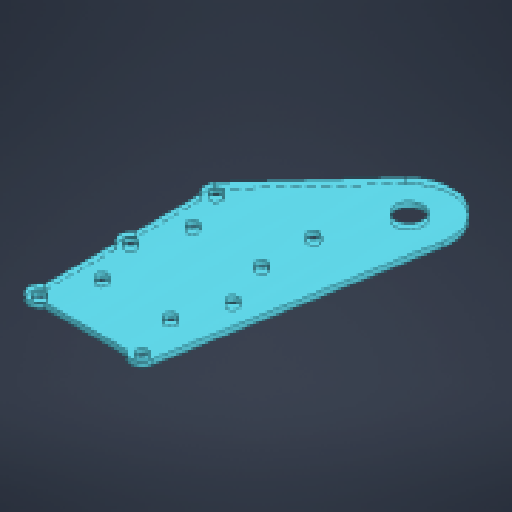
# Autodesk Inventor part: femur_support_steel
Saved by Autodesk Inventor 2026 (Build 300175000, 175)
## iProperties
Created: 2026-04-24
Part Number: femur_support_steel
Material: Сталь
Document SubType Name: Modeling
Designer: user
Density: 7.85 g/cm^3
Appearance: Серо-синий
Mass: 237.917 g
Surface Area: 222.677 cm^2
Volume: 30.3078 cm^3
Author: user
Autodesk Inventor part; units mm, degrees
ref_plane "YZ Plane" through (0, 0, 0) normal (1, 0, 0) x (0, 1, 0)
ref_plane "XZ Plane" through (0, 0, 0) normal (0, 1, 0) x (-1, 0, 0)
ref_plane "XY Plane" through (0, 0, 0) normal (0, 0, 1) x (1, 0, 0)
sketch "Эскиз1" plane through (0, 0, 0) normal (0, 1, 0) x (-1, 0, 0)
  circle A0 centre (41.8656, -145.8142) radius 7.75
  line L0 (111.6413, -108.8142) -> (38.7953, -108.8142) construction
  line L1 (76.8656, 21.9817) -> (76.8656, -112.0617)
  circle A1 centre (48.8156, -8.8142) radius 3.05
  circle A2 centre (57.9156, -33.8142) radius 3.05
  circle A3 centre (48.8156, -58.8142) radius 3.05
  circle A4 centre (57.9156, -83.8142) radius 3.05
  circle A5 centre (95.8156, -83.8142) radius 3.05
  circle A6 centre (104.9156, -58.8142) radius 3.05
  circle A7 centre (95.8156, -33.8142) radius 3.05
  circle A8 centre (104.9156, -8.8142) radius 3.05
  arc A9 (54.0984, -5.7642) -> (42.7519, -8.1498) centre (48.8156, -8.8142) ccw
  arc A10 (107.9656, -14.0969) -> (99.6329, -5.7642) centre (104.9156, -8.8142) ccw
  arc A11 (107.9656, -64.0969) -> (107.9656, -53.5314) centre (104.9156, -58.8142) ccw
  line L2 (107.9656, -102.9344) -> (107.9656, -64.0969)
  line L3 (107.9656, -53.5314) -> (107.9656, -14.0969)
  line L4 (99.6329, -5.7642) -> (54.0984, -5.7642)
  line L5 (32.6597, -100.2644) -> (42.7519, -8.1498)
  circle A12 centre (41.8656, -145.8142) radius 15 construction
  line L6 (101.8656, -108.8142) -> (101.8656, -72.3334) construction
  line L7 (101.8656, -108.8142) -> (26.8312, -181.1395) construction
  line L8 (51.8656, -108.8142) -> (51.8656, -72.3334) construction
  line L9 (95.7259, -114.7322) -> (107.9656, -102.9344)
  line L10 (95.7259, -114.7322) -> (98.5019, -117.6122)
  arc A13 (98.4405, -120.4492) -> (98.5019, -117.6122) centre (97.0619, -119.0002) ccw
  circle A14 centre (41.8656, -145.8142) radius 45 construction
  circle A15 centre (77.839, -118.7786) radius 5.05
  circle A16 centre (5.8923, -172.8497) radius 5.05
  arc A17 (-4.5085, -167.9431) -> (7.7127, -184.2047) centre (5.8923, -172.8497) ccw
  line L11 (-4.5085, -167.9431) -> (12.4721, -131.9479)
  line L12 (26.8312, -181.1395) -> (30.2073, -177.8853)
  line L13 (32.4723, -180.2351) -> (30.2073, -177.8853)
  arc A18 (47.0104, -177.9044) -> (71.2591, -159.6804) centre (41.8656, -145.8142) ccw
  arc A19 (21.5713, -120.4293) -> (12.4721, -131.9479) centre (41.8656, -145.8142) ccw
  line L14 (98.4405, -120.4492) -> (86.4967, -131.9617)
  line L15 (71.2591, -159.6804) -> (80.184, -140.7616)
  arc A20 (21.5713, -120.4293) -> (32.6597, -100.2644) centre (2.8381, -96.9971) ccw
  line L16 (7.7127, -184.2047) -> (26.8312, -181.1395)
  line L17 (32.4723, -180.2351) -> (47.0104, -177.9044)
  arc A21 (86.4967, -131.9617) -> (80.184, -140.7616) centre (107.3164, -153.5612) ccw
  point P0 (0, 0)
  point P1 (99.8898, -119.0521)
  point P2 (31.026, -115.1751)
  point P3 (82.5329, -135.7824)
  dimension "d4" = 37.9
  dimension "d5" = 56.1
  dimension "d6" = 6.1
  dimension "d7" = 50
  dimension "d8" = 50
  dimension "d9" = 25
  dimension "d10" = 50
  dimension "d11" = 37.9
  dimension "d12" = 56.1
  dimension "d15" = 35
  dimension "d16" = 37
  dimension "d17" = 15.5
  dimension "d20" = 12.2
  dimension "d21" = 12.2
  dimension "d24" = 3.05
  dimension "d26" = 30
  dimension "d29" = 50
  dimension "d33" = 10.1
  dimension "d36" = 360
  dimension "d38" = 90
  dimension "d40" = 9.5
  dimension "d42" = 32.5
  dimension "d44" = 23
  dimension "d45" = 6
  dimension "d47" = 11.5
  dimension "d48" = 30
  dimension "d49" = 17
  dimension "d50" = 91
  dimension "d51" = 30
  constraints: 36 end point, 21 centre point, 19 point on circle, 15 tangent, 11 point on line, 9 equal radius, 7 coincident, 4 horizontal alignment, 4 perpendicular, 4 vertical alignment, 2 symmetric about line, 2 vertical, 1 horizontal, 1 parallel, 9 other
  measures "d4" distance of A5.centre A4.centre
  measures "d5" distance of A8.centre A1.centre
  measures "d6" diameter of A1
  measures "d7" distance from line of A3.centre L0
  measures "d8" distance of A1.centre A3.centre
  measures "d9" distance from line of L0 A4.centre
  measures "d10" distance of A2.centre A4.centre
  measures "d11" diameter of A2.centre L1
  measures "d12" diameter of A1.centre L1
  measures "d15" distance from line of A0.centre L1
  measures "d16" distance from line of L0 A0.centre
  measures "d17" diameter of A0
  measures "d20" diameter of A10
  measures "d21" diameter of A11
  measures "d24" distance from line of L4 A8.centre
  measures "d26" diameter of A12
  measures "d29" diameter of L6 L1
  measures "d33" diameter of A15
  measures "d38" distance of A16.centre A15.centre
  measures "d40" distance from line of L7 A15.centre
  measures "d42" radius of A19
  measures "d44" diameter of A17
  measures "d45" distance between parallel lines of L14 L7
  measures "d47" distance from line of L15 A15.centre
  measures "d48" radius of A20
  measures "d49" distance from line of L10 L2.start
  measures "d50" distance between parallel lines of L10 L13
  measures "d51" radius of A21
extrude "Выдавливание1" add sketch "Эскиз1" along normal blind 3
equation "\"d4\" = -d_main_screw_holes + hight_profile_femur - 2 * thickness_profile_femur"
equation "\"d5\" = hight_profile_femur + d_main_screw_holes"
equation "\"d6\" = d_main_screw_holes"
equation "\"d11\" = -d_main_screw_holes + hight_profile_femur - 2 * thickness_profile_femur"
equation "\"d12\" = hight_profile_femur + d_main_screw_holes"
equation "\"d15\" = width_shaft_shift"
equation "\"d20\" = 2 * d_main_screw_holes"
equation "\"d21\" = 2 * d_main_screw_holes"
equation "\"d24\" = 0.5 * d_main_screw_holes"
equation "\"d29\" = width_profile_femur"
equation "\"d2\" = thickness_steel"
equation "\"tolerance_plazma\" = 0.1"
equation "\"thickness_steel\" = 3"
equation "\"d_main_screw_holes\" = 6.1"
equation "\"d_main_shaft\" = 15"
equation "\"thickness_profile_tibea\" = 3"
equation "\"hight_shaft_shift\" = 37"
equation "\"thickness_profile_femur\" = 3"
equation "\"width_profile_femur\" = 50"
equation "\"width_shaft_shift\" = 35"
equation "\"hight_profile_femur\" = 50"
equation "\"width_flattened_surface\" = 12"
